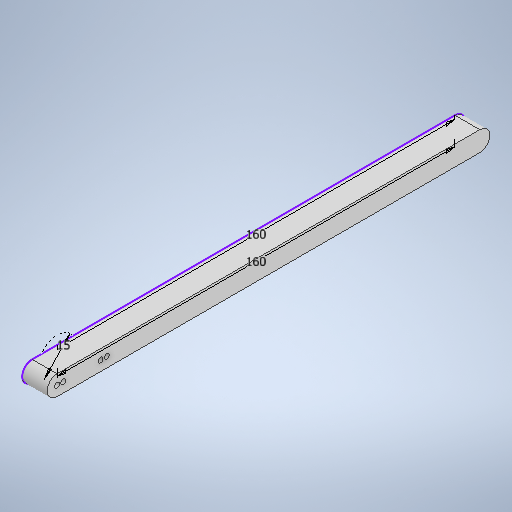
# Autodesk Inventor part: Leg
Saved by Autodesk Inventor 2025 (Build 290162000, 162)
## iProperties
Created: 2025-12-07
Part Number: Leg
Material: Типовые
Document SubType Name: Modeling
Designer: Admin
Density: 1 g/cm^3
Appearance: По умолчанию
Author: Admin
Autodesk Inventor part; units mm, degrees
ref_plane "YZ Plane" through (0, 0, 0) normal (1, 0, 0) x (0, 1, 0)
ref_plane "XZ Plane" through (0, 0, 0) normal (0, 1, 0) x (-1, 0, 0)
ref_plane "XY Plane" through (0, 0, 0) normal (0, 0, 1) x (1, 0, 0)
sketch "Эскиз1" plane through (0, 0, 0) normal (1, 0, 0) x (0, 1, 0)
  circle A0 centre (0, 0) radius 7.5 construction
  line L0 (4, 0) -> (4, -160)
  line L1 (-4, 0) -> (-4, -160)
  arc A1 (-4, -160) -> (4, -160) centre (0, -160) ccw
  line L2 (4, 0) -> (4, 10)
  line L3 (-4, 10) -> (-4, 0)
  arc A2 (4, 10) -> (-4, 10) centre (0, 10) ccw
  point P0 (0, -7.5)
  point P1 (0, -10)
  point P2 (0, 7.5)
  dimension "d0" = 15
  dimension "d2" = 160
  dimension "d3" = 160
  constraints: 8 end point, 6 point on circle, 3 centre point, 3 vertical, 2 coincident, 1 parallel
  measures "d0" diameter of A0
  measures "d2" distance of L0.start L0.end
  measures "d3" distance of L1.start L1.end
extrude "Выдавливание1" add sketch "Эскиз1" along normal blind 10
hole "Отверстие1" at (0, 0, -7.5) at (0, 0, -10) at (0, 0, 7.5) at (0, 0, 10) direction (1, 0, 0) diameter 2 end through all counterbore diameter 5 counterbore depth 5
